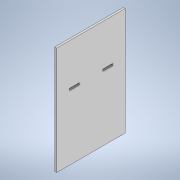
# Autodesk Inventor part: mount_slottedPanel
Saved by Autodesk Inventor 2020 (Build 240168000, 168)
## iProperties
Created: 2020-05-29
Part Number: mount_slottedPanel
Material: Generic
Document SubType Name: Modeling
Designer: lu0248
Density: 1 g/cm^3
Appearance: Default
Author: lu0248
Autodesk Inventor part; units mm, degrees
ref_plane "YZ Plane" through (0, 0, 0) normal (1, 0, 0) x (0, 1, 0)
ref_plane "XZ Plane" through (0, 0, 0) normal (0, 1, 0) x (-1, 0, 0)
ref_plane "XY Plane" through (0, 0, 0) normal (0, 0, 1) x (1, 0, 0)
sketch "Sketch1" plane through (0, 0, 0) normal (1, 0, 0) x (0, 1, 0)
  line L0 (550, 175) -> (0, 175)
  line L1 (0, 175) -> (0, -175)
  line L2 (0, -175) -> (550, -175)
  line L3 (550, -175) -> (550, 175)
  point P0 (0, 0)
  point P1 (0, 0)
  dimension "d0" = 550
  dimension "d1" = 350
  dimension "d2" = 175
  dimension "d3" = 0
  constraints: 8 end point, 2 parallel, 1 horizontal, 1 midpoint, 1 perpendicular
  measures "d0" distance of L0.start L0.end
  measures "d1" distance of L2.end L0.start
  measures "d2" distance from line of L0 point (0, 0)
  measures "d3" distance from line of point (0, 0) L1
extrude "Extrusion1" add sketch "Sketch1" along normal blind 10
sketch "Sketch2" plane through (10, 0, 0) normal (1, 0, 0) x (0, 0, -1)
  line L0 (-110, 340) -> (-60, 340)
  line L1 (-60, 340) -> (-60, 330)
  line L2 (-110, 330) -> (-110, 340)
  line L3 (110, 340) -> (60, 340)
  line L4 (60, 340) -> (60, 330)
  line L5 (60, 330) -> (110, 330)
  line L6 (110, 330) -> (110, 340)
  line L7 (175, 550) -> (-175, 550) projected
  line L8 (-110, 330) -> (-60, 330)
  point P0 (0, 0)
  dimension "d6" = 50
  dimension "d7" = 60
  dimension "d18" = 210
  dimension "d19" = 10
  dimension "d20" = 10
  dimension "d22" = 10
  dimension "d23" = 10
  dimension "d24" = 50
  dimension "d25" = 210
  dimension "d26" = 60
  constraints: 16 end point, 2 horizontal, 2 parallel, 1 perpendicular, 1 vertical
  measures "d6" distance of L0.start L0.end
  measures "d7" distance from line of point (0, 0) L1
  measures "d18" distance from line of L7 L0.end
  measures "d19" distance of L2.start L0.start
  measures "d20" distance of L0.end L1.end
  measures "d22" distance of L3.end L4.end
  measures "d23" distance of L5.end L3.start
  measures "d24" distance of L3.start L3.end
  measures "d25" distance between parallel lines of L7 L3
  measures "d26" horizontal distance of point (0, 0) L3.end
extrude "Extrusion3" cut sketch "Sketch2" against normal blind 10
body "Solid1"
